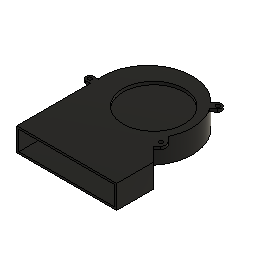
Fan - PVB120G12H-P01 v4 (Autodesk Fusion 360 design; units mm, degrees)
Autodesk Fusion 360 part; units mm, degrees
sketch "Esquisse1" plane through (0, 0, 0) normal (0, 0, 1) x (1, 0, 0)
  line L0 (0, 0) -> (98.3, 0)
  line L1 (98.3, 0) -> (98.3, 36.6)
  line L2 (98.3, 36.6) -> (77.8168, 56.6)
  arc A0 (77.8168, 56.6) -> (0, 84.75) centre (44, 84.75) ccw
  line L3 (0, 84.75) -> (0, 0)
  circle A1 centre (50.69, 84) radius 30.15
  point P0 (44, 128.75)
  point P1 (80.84, 84)
  point P2 (88, 84.75)
  point P3 (50.69, 114.15)
  dimension "d1" = 98.3
  dimension "d2" = 36.6
  dimension "d3" = 128.75
  dimension "d4" = 44
  dimension "d5" = 56.6
  dimension "d6" = 60.3
  dimension "d23" = 7.16
  dimension "d24" = 14.6
  constraint coincident L0.start L3.end
  constraint horizontal L0
  constraint perpendicular L0 L1
  constraint vertical L3
  constraint tangent A0 L3
  constraint coincident A0 P0
  constraint vertical A0.centre P0
  constraint coincident A1 P1
  constraint horizontal A1.centre P1
  constraint coincident A0 P2
  constraint horizontal A0.centre P2
  constraint coincident A1 P3
  constraint vertical A1.centre P3
  measures "d1" distance of L0.start L0.end
  measures "d2" distance of L0.end L1.end
  measures "d3" distance of L0 P0
  measures "d4" radius of A0
  measures "d5" distance of L0 L2.end
  measures "d6" diameter of A1
  measures "d23" horizontal distance of P1 P2
  measures "d24" vertical distance of P0 P3
extrude "Extrusion1" add sketch "Esquisse1" along normal blind 23.06 contours L0 L1 L2 A0 L3 | A1
extrude "Extrusion2" cut sketch "Esquisse1" against normal blind 3 from surface at 23.06 contours A1
shell "Coque1" thickness 2 removed faces 1 at (32.7667, 0, 7.6867)
ref_plane "Plan de construction1" through (49.3725, 68.154, 23.06) normal (0, 0, 1) x (1, 0, 0)
sketch "Esquisse2" plane through (0, 0, 23.06) normal (0, 0, 1) x (1, 0, 0)
  circle A0 centre (84.6158, 57.1208) radius 1.95
  circle A1 centre (81.8543, 116.0561) radius 1.95
  circle A2 centre (-4.3677, 76.1716) radius 1.95
  line L0 (81.8543, 116.0561) -> (84.6158, 57.1208) construction
  line L1 (84.6158, 57.1208) -> (-4.3677, 76.1716) construction
  line L2 (81.8543, 116.0561) -> (-4.3677, 76.1716) construction
  circle A3 centre (44, 84.75) radius 49.1225 construction
  arc A4 (77.8168, 56.6) -> (0, 84.75) centre (44, 84.75) ccw construction
  circle A5 centre (84.6158, 57.1208) radius 5.1225
  line L3 (98.3, 36.6) -> (77.8168, 56.6) construction
  line L4 (84.7023, 49.877) -> (91.8596, 57.2072)
  line L5 (91.8596, 57.2072) -> (83.5013, 65.3684)
  line L6 (80.2019, 109.7584) -> (84.2761, 113.1278)
  arc A6 (84.2761, 113.1278) -> (79.4325, 118.9844) centre (81.8543, 116.0561) ccw
  line L7 (79.4325, 118.9844) -> (75.3584, 115.615)
  line L8 (0, 72.3716) -> (-4.3677, 72.3716)
  arc A7 (-4.3677, 79.9716) -> (-4.3677, 72.3716) centre (-4.3677, 76.1716) ccw
  line L9 (-4.3677, 79.9716) -> (0.2602, 79.9716)
  line L10 (81.8543, 116.0561) -> (44, 84.75) construction
  line L11 (44, 84.75) -> (84.6158, 57.1208) construction
  arc A8 (77.8168, 56.6) -> (0, 84.75) centre (44, 84.75) ccw
  line L12 (0, 84.75) -> (0, 0)
  line L13 (98.3, 36.6) -> (77.8168, 56.6)
  dimension "d15" = 3.9
  dimension "d16" = 59
  dimension "d17" = 95
  dimension "d18" = 91
  dimension "d19" = 7.6
  dimension "d20" = 7.6
  constraint coincident A0.centre L0.end
  constraint coincident A2.centre L1.end
  constraint coincident A1.centre L0.start
  constraint equal A0 A1
  constraint equal A0 A2
  constraint coincident A0.centre A3
  constraint coincident A1.centre A3
  constraint coincident A2.centre A3
  constraint concentric A3 A4
  constraint concentric A0 A5
  constraint tangent A4 A5
  constraint tangent A5 L3
  constraint coincident L3 L4.start
  constraint coincident A4 L5.end
  constraint perpendicular L4 L5
  constraint perpendicular L3 L4
  constraint coincident A4 L6.start
  constraint tangent L6 A6
  constraint coincident A4 L7.end
  constraint horizontal L8
  constraint tangent L8 A7
  constraint coincident A4 L9.end
  constraint tangent A7 L9
  constraint horizontal L9
  constraint parallel L6 L7
  constraint tangent A6 L7
  constraint coincident A3.centre A4.centre
  constraint parallel L7 L10
  constraint tangent A5 L4
  constraint tangent A5 L5
  measures "d15" diameter of A1
  measures "d16" distance of A1.centre A0.centre
  measures "d17" distance of A1.centre A2.centre
  measures "d18" distance of A0.centre A2.centre
  measures "d19" distance of L6 L7
  measures "d20" distance of L8.end A7.start
extrude "Extrusion3" add sketch "Esquisse2" against normal blind 2.8 contours A5 | A5 L5 A8 | A5 L4 L13 | A5 A8 L13 | L6 A6 L7 A8 | L8 A7 L9 L12
equation "d4 = ( 88 / 2 ) * 1 mm"
equation "d20 = d19"
